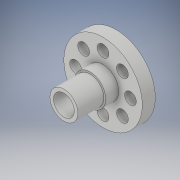
# Autodesk Inventor part: Hubnew
Saved by Autodesk Inventor 2019 (Build 230136000, 136)
## iProperties
Created: 2021-01-20
Part Number: Hubnew
Material: Generic
Document SubType Name: Modeling
Designer: Admin
Density: 1 g/cm^3
Appearance: Default
Author: Admin
Autodesk Inventor part; units mm, degrees
ref_plane "YZ Plane" through (0, 0, 0) normal (1, 0, 0) x (0, 1, 0)
ref_plane "XZ Plane" through (0, 0, 0) normal (0, 1, 0) x (-1, 0, 0)
ref_plane "XY Plane" through (0, 0, 0) normal (0, 0, 1) x (1, 0, 0)
sketch "Sketch1" plane through (0, 0, 0) normal (0, 0, 1) x (1, 0, 0)
  circle A0 centre (0, 0) radius 15
  circle A1 centre (0, 10.5) radius 2.25
  circle A2 centre (-7.4246, 7.4246) radius 2.25
  circle A3 centre (-10.5, 0) radius 2.25
  circle A4 centre (-7.4246, -7.4246) radius 2.25
  circle A5 centre (0, -10.5) radius 2.25
  circle A6 centre (7.4246, -7.4246) radius 2.25
  circle A7 centre (10.5, 0) radius 2.25
  circle A8 centre (7.4246, 7.4246) radius 2.25
  dimension "d0" = 30
  dimension "d2" = 4.5
  dimension "d5" = 360
  constraints: 9 centre point, 1 coincident, 17 other
  measures "d0" diameter of A0
  measures "d2" diameter of A1
extrude "Extrusion1" add sketch "Sketch1" along normal blind 5
sketch "Sketch2" plane through (0, 0, 5) normal (0, 0, 1) x (1, 0, 0)
  circle A0 centre (0, 0) radius 4
  circle A1 centre (0, 0) radius 5.3414
  circle A2 centre (0, 0) radius 6
  dimension "d9" = 8
  constraints: 3 centre point, 3 coincident
  measures "d9" diameter of A0
extrude "Extrusion2" add sketch "Sketch2" along normal blind 5 contours A2
extrude "Extrusion3" add sketch "Sketch2" along normal blind 15 contours A1
extrude "Extrusion4" cut sketch "Sketch2" against normal blind 21 contours A0
body "Solid1"
